Autodesk Fusion 360 part; units mm, degrees
(part 2 of 2)
  spline S18 degree 5 poles (-6.5449, 6.7429) (-6.5503, 6.7485) (-6.5613, 6.7594) (-6.5783, 6.7752) (-6.602, 6.7952) (-6.633, 6.8186) (-6.6649, 6.8409) (-6.6975, 6.8626) (-6.7305, 6.8839) (-6.7637, 6.905) (-6.7971, 6.9257) (-6.8309, 6.9462) (-6.8651, 6.9661) (-6.8998, 6.9854) (-6.9349, 7.0042) (-6.9705, 7.0225) (-7.0064, 7.0403) (-7.0427, 7.0577) (-7.0792, 7.0748) (-7.116, 7.0916) (-7.153, 7.108) (-7.1903, 7.1241) (-7.2279, 7.1398) (-7.2657, 7.1551) (-7.3038, 7.1701) (-7.3422, 7.1847) (-7.3809, 7.1989) (-7.4197, 7.2128) (-7.4588, 7.2264) (-7.4982, 7.2396) (-7.5377, 7.2526) (-7.5775, 7.2652) (-7.6174, 7.2774) (-7.6576, 7.2894) (-7.698, 7.301) (-7.7386, 7.3123) (-7.7793, 7.3233) (-7.8203, 7.334) (-7.8615, 7.3444) (-7.9028, 7.3544) (-7.9443, 7.3642) (-7.986, 7.3737) (-8.0279, 7.3828) (-8.07, 7.3916) (-8.1122, 7.4002) (-8.1545, 7.4084) (-8.1971, 7.4164) (-8.2398, 7.424) (-8.2826, 7.4313) (-8.3256, 7.4384) (-8.3688, 7.4451) (-8.4121, 7.4516) (-8.4555, 7.4577) (-8.4991, 7.4636) (-8.5429, 7.4692) (-8.5867, 7.4745) (-8.6307, 7.4795) (-8.6749, 7.4842) (-8.7191, 7.4886) (-8.7635, 7.4927) (-8.808, 7.4965) (-8.8527, 7.5001) (-8.8974, 7.5034) (-8.9423, 7.5063) (-8.9873, 7.509) (-9.0324, 7.5114) (-9.0777, 7.5136) (-9.123, 7.5154) (-9.1684, 7.5169) (-9.214, 7.5182) (-9.2596, 7.5192) (-9.2962, 7.5198) (-9.3237, 7.52) (-9.3421, 7.5202) (-9.3513, 7.5202) knots 0 0 0 0 0 0 0.01428571 0.02857143 0.04285714 0.05714286 0.07142857 0.08571429 0.1 0.11428571 0.12857143 0.14285714 0.15714286 0.17142857 0.18571429 0.2 0.21428571 0.22857143 0.24285714 0.25714286 0.27142857 0.28571429 0.3 0.31428571 0.32857143 0.34285714 0.35714286 0.37142857 0.38571429 0.4 0.41428571 0.42857143 0.44285714 0.45714286 0.47142857 0.48571429 0.5 0.51428571 0.52857143 0.54285714 0.55714286 0.57142857 0.58571429 0.6 0.61428571 0.62857143 0.64285714 0.65714286 0.67142857 0.68571429 0.7 0.71428571 0.72857143 0.74285714 0.75714286 0.77142857 0.78571429 0.8 0.81428571 0.82857143 0.84285714 0.85714286 0.87142857 0.88571429 0.9 0.91428571 0.92857143 0.94285714 0.95714286 0.97142857 0.98571429 1 1 1 1 1 1
  arc A38 (-9.3513, 7.5202) -> (-10.0419, 6.5697) centre (0, 0) ccw
  spline S19 degree 5 poles (-10.0419, 6.5697) (-10.039, 6.561) (-10.0332, 6.5436) (-10.0244, 6.5175) (-10.0126, 6.4829) (-9.9975, 6.4398) (-9.9822, 6.3968) (-9.9667, 6.3541) (-9.951, 6.3115) (-9.935, 6.2692) (-9.9187, 6.227) (-9.9023, 6.1851) (-9.8856, 6.1433) (-9.8686, 6.1017) (-9.8515, 6.0604) (-9.8341, 6.0192) (-9.8164, 5.9783) (-9.7986, 5.9376) (-9.7804, 5.897) (-9.7621, 5.8567) (-9.7435, 5.8166) (-9.7247, 5.7768) (-9.7056, 5.7371) (-9.6864, 5.6977) (-9.6668, 5.6585) (-9.6471, 5.6196) (-9.6271, 5.5808) (-9.6069, 5.5424) (-9.5864, 5.5041) (-9.5657, 5.4661) (-9.5448, 5.4283) (-9.5236, 5.3908) (-9.5022, 5.3536) (-9.4806, 5.3166) (-9.4587, 5.2799) (-9.4366, 5.2434) (-9.4142, 5.2072) (-9.3917, 5.1712) (-9.3688, 5.1356) (-9.3458, 5.1002) (-9.3225, 5.0651) (-9.299, 5.0303) (-9.2752, 4.9957) (-9.2511, 4.9615) (-9.2269, 4.9276) (-9.2024, 4.894) (-9.1776, 4.8607) (-9.1526, 4.8277) (-9.1274, 4.795) (-9.1019, 4.7627) (-9.0762, 4.7307) (-9.0502, 4.699) (-9.0239, 4.6678) (-8.9973, 4.6369) (-8.9705, 4.6064) (-8.9435, 4.5763) (-8.9162, 4.5465) (-8.8886, 4.517) (-8.8608, 4.4879) (-8.8328, 4.4593) (-8.8044, 4.4311) (-8.7757, 4.4035) (-8.7466, 4.3765) (-8.7171, 4.3501) (-8.6872, 4.3243) (-8.6571, 4.2989) (-8.6268, 4.2738) (-8.5964, 4.2491) (-8.5657, 4.2248) (-8.5346, 4.2013) (-8.5027, 4.179) (-8.4764, 4.1627) (-8.4561, 4.1514) (-8.4423, 4.1443) (-8.4354, 4.1409) knots -1 -1 -1 -1 -1 -1 -0.98571429 -0.97142857 -0.95714286 -0.94285714 -0.92857143 -0.91428571 -0.9 -0.88571429 -0.87142857 -0.85714286 -0.84285714 -0.82857143 -0.81428571 -0.8 -0.78571429 -0.77142857 -0.75714286 -0.74285714 -0.72857143 -0.71428571 -0.7 -0.68571429 -0.67142857 -0.65714286 -0.64285714 -0.62857143 -0.61428571 -0.6 -0.58571429 -0.57142857 -0.55714286 -0.54285714 -0.52857143 -0.51428571 -0.5 -0.48571429 -0.47142857 -0.45714286 -0.44285714 -0.42857143 -0.41428571 -0.4 -0.38571429 -0.37142857 -0.35714286 -0.34285714 -0.32857143 -0.31428571 -0.3 -0.28571429 -0.27142857 -0.25714286 -0.24285714 -0.22857143 -0.21428571 -0.2 -0.18571429 -0.17142857 -0.15714286 -0.14285714 -0.12857143 -0.11428571 -0.1 -0.08571429 -0.07142857 -0.05714286 -0.04285714 -0.02857143 -0.01428571 0 0 0 0 0 0
  line L19 (-8.4354, 4.1409) -> (-7.6212, 3.7403)
  arc A39 (-7.1196, 2.5104) -> (-7.6212, 3.7403) centre (-8.0626, 2.843) ccw
  circle A40 centre (0, 0) radius 17.5
  dimension "d9" = 35
  constraint concentric A0 A40
  measures "d9" diameter of A40
extrude "Extrude3" add sketch "Sketch1 (2)" along normal blind 7 contours A0 A1 L0 S0 A2 S1 L1 A3 A4 A5 L2 S2 A6 S3 L3 A7 A8 A9 L4 S4 A10 S5 L5 A11 A12 A13 L6 S6 A14 S7 L7 A15 A16 A17 L8 S8 A18 S9 L9 A19 A20 A21 L10 S10 A22 S11 L11 A23 A24 A25 L12 S12 A26 S13 L13 A27 A28 A29 L14 S14 A30 S15 L15 A31 A32 A33 L16 S16 A34 S17 L17 A35 A36 A37 L18 S18 A38 S19 L19 A39 | A40 bodies 1 in component "Spur Gear (10 teeth)"
sketch "Sketch2 (2)" plane through (0, 0, 38) normal (0, 0, 1) x (-1, 0, 0)
  line L0 (-3.5, -6.0622) -> (3.5, -6.0622)
  line L1 (3.5, -6.0622) -> (7, 0)
  line L2 (7, 0) -> (3.5, 6.0622)
  line L3 (3.5, 6.0622) -> (-3.5, 6.0622)
  line L4 (-3.5, 6.0622) -> (-7, 0)
  line L5 (-7, 0) -> (-3.5, -6.0622)
  circle A0 centre (0, 0) radius 5.75
extrude "Extrude4" cut sketch "Sketch2 (2)" against normal blind 31 contours L0 L1 L2 L3 L4 L5 | A0 bodies 1 in component "Spur Gear (10 teeth)"
extrude "Extrude5" cut 1 faces at (-2.3777, 0.694, 0) along direction (0, 0, 1) blind 7 on bodies 1 bodies 1 in component "Spur Gear (10 teeth)"
extrude "Extrude6" add 1 faces at (8.7557, 4.5517, 14) along direction (0, 0, 1) blind 2 on bodies 1 bodies 1 in component "Spur Gear (10 teeth)"
sketch "Sketch3 (2)" plane through (0, 0, 7) normal (0, 0, -1) x (1, 0, 0)
  line L0 (-3.5, 6.0622) -> (3.5, 6.0622)
  line L1 (3.5, 6.0622) -> (7, 0)
  line L2 (7, 0) -> (3.5, -6.0622)
  line L3 (3.5, -6.0622) -> (-3.5, -6.0622)
  line L4 (-3.5, -6.0622) -> (-7, 0)
  line L5 (-7, 0) -> (-3.5, 6.0622)
  circle A0 centre (0, 0) radius 17.5
  arc A1 (-44.2503, 36.7173) -> (-43.1721, 30.6989) centre (-41.1721, 34.163) ccw
  line L6 (-26.1836, 58.9803) -> (-29.7874, 57.2447)
  line L7 (-37.9866, 52.1658) -> (-38.2509, 52.5535)
  line L8 (7.3412, 1.535) -> (14.1913, -2.4199)
  arc A2 (44.2503, 36.7173) -> (-44.2503, 36.7173) centre (0, 0) ccw
  arc A3 (-2.3412, -7.1252) -> (2.3412, -7.1252) centre (0, 0) ccw
  line L9 (17.1006, -62.224) -> (20.9229, -61.0449)
  line L10 (37.9866, 52.1658) -> (34.6817, 54.419)
  arc A4 (57.265, -30.7526) -> (59.7475, -25.5977) centre (0, 0) ccw
  line L11 (-7.6356, -64.0777) -> (-7.7055, -64.5417)
  line L12 (-34.6817, -54.419) -> (-34.946, -54.8067)
  arc A5 (2, -64.9692) -> (7.7055, -64.5417) centre (0, 0) ccw
  arc A6 (-48.1721, 22.0387) -> (-53.9232, 19.9633) centre (-50.1721, 18.5746) ccw
  line L13 (56.8586, 30.5179) -> (54.8586, 33.9821)
  arc A7 (55.265, 34.2167) -> (52.042, 38.944) centre (0, 0) ccw
  arc A8 (9.1913, -11.0801) -> (14.6554, -9.616) centre (11.1913, -7.616) ccw
  line L14 (-38.2509, -52.5535) -> (-37.9866, -52.1658)
  arc A9 (64.6381, 6.8496) -> (63.7854, 12.5072) centre (0, 0) ccw
  line L15 (29.7874, -57.2447) -> (29.991, -57.6675)
  line L16 (42.405, -48.6422) -> (45.3372, -45.9215)
  line L17 (-45.6564, -46.2655) -> (-45.3372, -45.9215)
  line L18 (52.042, 38.944) -> (51.6751, 38.6514)
  line L19 (-29.7874, -57.2447) -> (-26.1836, -58.9803)
  line L20 (64.1702, 6.8145) -> (64.6381, 6.8496)
  line L21 (-26.1836, -58.9803) -> (-26.3872, -59.403)
  arc A10 (5, -52.7376) -> (9.6729, -56.6806) centre (9, -52.7376) ccw
  line L22 (51.6751, -38.6514) -> (52.042, -38.944)
  line L23 (-54.8586, -33.9821) -> (-55.265, -34.2167)
  line L24 (15.6554, -7.884) -> (14.6554, -9.616)
  arc A11 (21.0612, -61.4933) -> (26.3872, -59.403) centre (0, 0) ccw
  line L25 (-54.8586, 33.9821) -> (-56.8586, 30.5179)
  line L26 (-11.6608, -63.9455) -> (-11.5909, -63.4815)
  arc A12 (-42.7242, -48.9862) -> (-38.2509, -52.5535) centre (0, 0) ccw
  line L27 (-42.405, -48.6422) -> (-42.7242, -48.9862)
  arc A13 (-49.548, -42.0713) -> (-45.6564, -46.2655) centre (0, 0) ccw
  line L28 (49.1812, 41.7788) -> (49.548, 42.0713)
  line L29 (-37.9866, -52.1658) -> (-34.6817, -54.419)
  arc A14 (-23.6426, 19.4236) -> (-18.8944, 19.9813) centre (-21.6426, 22.8877) ccw
  line L30 (2, -64.5) -> (2, -64.9692)
  arc A15 (-9.6729, -56.6806) -> (-5, -52.7376) centre (-9, -52.7376) ccw
  line L31 (26.1836, -58.9803) -> (29.7874, -57.2447)
  arc A16 (-17.2389, -62.6723) -> (-11.6608, -63.9455) centre (0, 0) ccw
  arc A17 (-34.946, -54.8067) -> (-29.991, -57.6675) centre (0, 0) ccw
  line L32 (-49.1812, -41.7788) -> (-49.548, -42.0713)
  arc A18 (52.042, -38.944) -> (55.265, -34.2167) centre (0, 0) ccw
  arc A19 (43.1721, 30.6989) -> (44.2503, 36.7173) centre (41.1721, 34.163) ccw
  arc A20 (61.2088, -21.8742) -> (62.8953, -16.4069) centre (0, 0) ccw
  arc A21 (62.8953, 16.4069) -> (61.2088, 21.8742) centre (0, 0) ccw
  line L33 (59.3107, -25.4262) -> (60.772, -21.7027)
  line L34 (5, -52.7376) -> (5, -30.1869)
  line L35 (61.2088, 21.8742) -> (60.772, 21.7027)
  line L36 (17.2389, -62.6723) -> (17.1006, -62.224)
  line L37 (7.7055, -64.5417) -> (7.6356, -64.0777)
  line L38 (64.6381, -6.8496) -> (64.1702, -6.8145)
  line L39 (42.405, 48.6422) -> (42.7242, 48.9862)
  line L40 (45.3372, -45.9215) -> (45.6564, -46.2655)
  arc A22 (-7.7055, -64.5417) -> (-2, -64.9692) centre (0, 0) ccw
  line L41 (64.1702, -6.8145) -> (64.4691, -2.8257)
  line L42 (62.8953, -16.4069) -> (62.4378, -16.3025)
  arc A23 (7.8571, -26.3537) -> (5, -30.1869) centre (9, -30.1869) ccw
  line L43 (62.4378, -16.3025) -> (63.3279, -12.4027)
  line L44 (-63.7854, -12.5072) -> (-63.3279, -12.4027)
  arc A24 (5, 13.5) -> (1, 17.5) centre (1, 13.5) ccw
  line L45 (26.1836, 58.9803) -> (26.3872, 59.403)
  line L46 (20.9229, -61.0449) -> (21.0612, -61.4933)
  arc A25 (26.3872, 59.403) -> (21.0612, 61.4933) centre (0, 0) ccw
  line L47 (-34.6817, 54.419) -> (-37.9866, 52.1658)
  arc A26 (-57.265, 30.7526) -> (-59.7475, 25.5977) centre (0, 0) ccw
  arc A27 (-62.8953, -16.4069) -> (-61.2088, -21.8742) centre (0, 0) ccw
  line L48 (-64.937, -2.8607) -> (-64.4691, -2.8257)
  arc A28 (-64.6381, -6.8496) -> (-63.7854, -12.5072) centre (0, 0) ccw
  line L49 (-23.6426, 19.4236) -> (-43.1721, 30.6989)
  line L50 (64.4691, 2.8257) -> (64.1702, 6.8145)
  arc A29 (-63.7854, 12.5072) -> (-64.6381, 6.8496) centre (0, 0) ccw
  arc A30 (-61.2088, 21.8742) -> (-62.8953, 16.4069) centre (0, 0) ccw
  arc A31 (29.991, -57.6675) -> (34.946, -54.8067) centre (0, 0) ccw
  arc A32 (15.6554, -7.884) -> (14.1913, -2.4199) centre (12.1913, -5.884) ccw
  line L51 (2, 64.9692) -> (2, 64.5)
  arc A33 (28.6426, 10.7633) -> (26.7515, 6.3723) centre (30.6426, 7.2992) ccw
  line L52 (5, 13.5) -> (5, 5.5902)
  line L53 (-63.3279, -12.4027) -> (-62.4378, -16.3025)
  line L54 (62.4378, 16.3025) -> (62.8953, 16.4069)
  line L55 (42.7242, -48.9862) -> (42.405, -48.6422)
  line L56 (-26.3872, 59.403) -> (-26.1836, 58.9803)
  arc A34 (7.7055, 64.5417) -> (2, 64.9692) centre (0, 0) ccw
  arc A35 (34.946, 54.8067) -> (29.991, 57.6675) centre (0, 0) ccw
  line L57 (21.0612, 61.4933) -> (20.9229, 61.0449)
  line L58 (7.6356, -64.0777) -> (11.5909, -63.4815)
  line L59 (55.265, -34.2167) -> (54.8586, -33.9821)
  line L60 (-62.4378, 16.3025) -> (-63.3279, 12.4027)
  line L61 (-20.9229, -61.0449) -> (-17.1006, -62.224)
  line L62 (-62.8953, 16.4069) -> (-62.4378, 16.3025)
  arc A36 (-38.2509, 52.5535) -> (-42.7242, 48.9862) centre (0, 0) ccw
  line L63 (-52.042, -38.944) -> (-51.6751, -38.6514)
  line L64 (-63.3279, 12.4027) -> (-63.7854, 12.5072)
  line L65 (-55.265, 34.2167) -> (-54.8586, 33.9821)
  line L66 (-56.8586, 30.5179) -> (-57.265, 30.7526)
  line L67 (49.1812, -41.7788) -> (51.6751, -38.6514)
  line L68 (-61.2088, -21.8742) -> (-60.772, -21.7027)
  line L69 (-64.4691, -2.8257) -> (-64.1702, -6.8145)
  line L70 (-17.1006, -62.224) -> (-17.2389, -62.6723)
  arc A37 (-5, -30.1869) -> (-7.8571, -26.3537) centre (-9, -30.1869) ccw
  line L71 (-2.3412, -7.1252) -> (-9.1913, -11.0801)
  line L72 (-29.991, -57.6675) -> (-29.7874, -57.2447)
  line L73 (43.1721, 30.6989) -> (23.6426, 19.4236)
  line L74 (-49.548, 42.0713) -> (-49.1812, 41.7788)
  arc A38 (-26.3872, -59.403) -> (-21.0612, -61.4933) centre (0, 0) ccw
  line L75 (11.5909, -63.4815) -> (11.6608, -63.9455)
  line L76 (11.6608, 63.9455) -> (11.5909, 63.4815)
  line L77 (-48.1721, 22.0387) -> (-28.6426, 10.7633)
  line L78 (56.8586, -30.5179) -> (57.265, -30.7526)
  line L79 (-62.4378, -16.3025) -> (-62.8953, -16.4069)
  line L80 (-64.1702, -6.8145) -> (-64.6381, -6.8496)
  line L81 (7.6356, 64.0777) -> (7.7055, 64.5417)
  line L82 (9.1913, -11.0801) -> (2.3412, -7.1252)
  line L83 (-51.6751, -38.6514) -> (-49.1812, -41.7788)
  arc A39 (-53.9232, 19.9633) -> (-9.6729, -56.6806) centre (0, 0) ccw
  line L84 (-14.1913, -2.4199) -> (-7.3412, 1.535)
  arc A40 (-64.937, 2.8607) -> (-64.937, -2.8607) centre (0, 0) ccw
  line L85 (-2, 64.5) -> (-2, 64.9692)
  line L86 (20.9229, 61.0449) -> (17.1006, 62.224)
  line L87 (-60.772, -21.7027) -> (-59.3107, -25.4262)
  arc A41 (-2, 64.9692) -> (-7.7055, 64.5417) centre (0, 0) ccw
  arc A42 (17.2389, 62.6723) -> (11.6608, 63.9455) centre (0, 0) ccw
  arc A43 (-55.265, -34.2167) -> (-52.042, -38.944) centre (0, 0) ccw
  line L88 (-59.7475, 25.5977) -> (-59.3107, 25.4262)
  arc A44 (-29.991, 57.6675) -> (-34.946, 54.8067) centre (0, 0) ccw
  arc A45 (64.937, -2.8607) -> (64.937, 2.8607) centre (0, 0) ccw
  line L89 (64.4691, -2.8257) -> (64.937, -2.8607)
  line L90 (-45.3372, -45.9215) -> (-42.405, -48.6422)
  line L91 (57.265, 30.7526) -> (56.8586, 30.5179)
  line L92 (63.3279, 12.4027) -> (62.4378, 16.3025)
  line L93 (34.6817, 54.419) -> (34.946, 54.8067)
  line L94 (60.772, -21.7027) -> (61.2088, -21.8742)
  line L95 (45.6564, 46.2655) -> (45.3372, 45.9215)
  line L96 (54.8586, -33.9821) -> (56.8586, -30.5179)
  line L97 (26.3872, -59.403) -> (26.1836, -58.9803)
  line L98 (45.3372, 45.9215) -> (42.405, 48.6422)
  arc A46 (49.548, 42.0713) -> (45.6564, 46.2655) centre (0, 0) ccw
  line L99 (64.937, 2.8607) -> (64.4691, 2.8257)
  arc A47 (11.6608, -63.9455) -> (17.2389, -62.6723) centre (0, 0) ccw
  arc A48 (38.2509, -52.5535) -> (42.7242, -48.9862) centre (0, 0) ccw
  arc A49 (45.6564, -46.2655) -> (49.548, -42.0713) centre (0, 0) ccw
  line L100 (34.6817, -54.419) -> (37.9866, -52.1658)
  line L101 (38.2509, 52.5535) -> (37.9866, 52.1658)
  line L102 (37.9866, -52.1658) -> (38.2509, -52.5535)
  arc A50 (53.9232, 19.9633) -> (48.1721, 22.0387) centre (50.1721, 18.5746) ccw
  arc A51 (63.7854, -12.5072) -> (64.6381, -6.8496) centre (0, 0) ccw
  arc A52 (42.7242, 48.9862) -> (38.2509, 52.5535) centre (0, 0) ccw
  line L103 (63.7854, 12.5072) -> (63.3279, 12.4027)
  arc A53 (59.7475, 25.5977) -> (57.265, 30.7526) centre (0, 0) ccw
  line L104 (59.7475, -25.5977) -> (59.3107, -25.4262)
  line L105 (60.772, 21.7027) -> (59.3107, 25.4262)
  line L106 (49.548, -42.0713) -> (49.1812, -41.7788)
  line L107 (63.3279, -12.4027) -> (63.7854, -12.5072)
  line L108 (34.946, -54.8067) -> (34.6817, -54.419)
  line L109 (51.6751, 38.6514) -> (49.1812, 41.7788)
  line L110 (59.3107, 25.4262) -> (59.7475, 25.5977)
  line L111 (54.8586, 33.9821) -> (55.265, 34.2167)
  arc A54 (-45.6564, 46.2655) -> (-49.548, 42.0713) centre (0, 0) ccw
  arc A55 (-21.0612, 61.4933) -> (-26.3872, 59.403) centre (0, 0) ccw
  arc A56 (-52.042, 38.944) -> (-55.265, 34.2167) centre (0, 0) ccw
  arc A57 (18.8944, 19.9813) -> (23.6426, 19.4236) centre (21.6426, 22.8877) ccw
  line L112 (-34.946, 54.8067) -> (-34.6817, 54.419)
  line L113 (-42.405, 48.6422) -> (-45.3372, 45.9215)
  line L114 (11.5909, 63.4815) -> (7.6356, 64.0777)
  arc A58 (18.8944, 19.9813) -> (-18.8944, 19.9813) centre (0, 0) ccw
  line L115 (-51.6751, 38.6514) -> (-52.042, 38.944)
  line L116 (-29.7874, 57.2447) -> (-29.991, 57.6675)
  arc A59 (9.6729, -56.6806) -> (53.9232, 19.9633) centre (0, 0) ccw
  line L117 (2, 64.5) -> (-2, 64.5)
  line L118 (-2, -64.5) -> (2, -64.5)
  line L119 (-1, 17.5) -> (1, 17.5)
  arc A60 (-26.7515, 6.3723) -> (-7.8571, -26.3537) centre (0, 0) ccw
  line L120 (-49.1812, 41.7788) -> (-51.6751, 38.6514)
  arc A61 (7.8571, -26.3537) -> (26.7515, 6.3723) centre (0, 0) ccw
  line L121 (-64.6381, 6.8496) -> (-64.1702, 6.8145)
  arc A62 (-5, 5.5902) -> (-7.3412, 1.535) centre (0, 0) ccw
  line L122 (-5, -30.1869) -> (-5, -52.7376)
  line L123 (17.1006, 62.224) -> (17.2389, 62.6723)
  line L124 (-7.7055, 64.5417) -> (-7.6356, 64.0777)
  line L125 (-20.9229, 61.0449) -> (-21.0612, 61.4933)
  arc A63 (-14.6554, -9.616) -> (-9.1913, -11.0801) centre (-11.1913, -7.616) ccw
  line L126 (29.991, 57.6675) -> (29.7874, 57.2447)
  line L127 (-14.6554, -9.616) -> (-15.6554, -7.884)
  line L128 (-42.7242, 48.9862) -> (-42.405, 48.6422)
  arc A64 (-14.1913, -2.4199) -> (-15.6554, -7.884) centre (-12.1913, -5.884) ccw
  line L129 (-59.3107, -25.4262) -> (-59.7475, -25.5977)
  line L130 (-17.1006, 62.224) -> (-20.9229, 61.0449)
  line L131 (-64.1702, 6.8145) -> (-64.4691, 2.8257)
  line L132 (-5, 5.5902) -> (-5, 13.5)
  line L133 (29.7874, 57.2447) -> (26.1836, 58.9803)
  line L134 (-11.5909, -63.4815) -> (-7.6356, -64.0777)
  arc A65 (-59.7475, -25.5977) -> (-57.265, -30.7526) centre (0, 0) ccw
  arc A66 (7.3412, 1.535) -> (5, 5.5902) centre (0, 0) ccw
  line L135 (-11.5909, 63.4815) -> (-11.6608, 63.9455)
  line L136 (-57.265, -30.7526) -> (-56.8586, -30.5179)
  line L137 (-45.3372, 45.9215) -> (-45.6564, 46.2655)
  line L138 (-59.3107, 25.4262) -> (-60.772, 21.7027)
  line L139 (-21.0612, -61.4933) -> (-20.9229, -61.0449)
  line L140 (-60.772, 21.7027) -> (-61.2088, 21.8742)
  line L141 (-2, -64.9692) -> (-2, -64.5)
  line L142 (28.6426, 10.7633) -> (48.1721, 22.0387)
  arc A67 (-1, 17.5) -> (-5, 13.5) centre (-1, 13.5) ccw
  line L143 (-56.8586, -30.5179) -> (-54.8586, -33.9821)
  line L144 (-17.2389, 62.6723) -> (-17.1006, 62.224)
  arc A68 (-26.7515, 6.3723) -> (-28.6426, 10.7633) centre (-30.6426, 7.2992) ccw
  arc A69 (-11.6608, 63.9455) -> (-17.2389, 62.6723) centre (0, 0) ccw
  line L145 (-7.6356, 64.0777) -> (-11.5909, 63.4815)
  line L146 (-64.4691, 2.8257) -> (-64.937, 2.8607)
extrude "Extrude1'" add sketch "Sketch3 (2)" along normal blind 6 separate body contours L0 L1 L2 L3 L4 L5 | A0 L8 A24 A32 L52 A66 | A0 L8 A3 A8 A24 A32 L52 L71 L82 L84 A62 A63 A64 L132 A66 A67 | A0 L84 A62 A64 L132 A67 | A0 A3 A8 L71 L82 A63 | L6 L7 L9 L10 A4 L11 L12 A5 L13 A7 L14 A9 L15 L16 L17 L18 L19 L20 L21 L22 L23 A11 L25 L26 A12 L27 A13 L28 L29 L30 L31 A16 A17 L32 A18 A20 A21 L33 L35 L36 L37 L38 L39 L40 A22 L41 L42 L43 L44 L45 L46 A25 L47 A26 A27 L48 A28 L50 A29 A30 A31 L51 L53 L54 L55 L56 A34 A35 L57 L58 L59 L60 L61 L62 A36 L63 L64 L65 L66 L67 L68 L69 L70 L72 L74 A38 L75 L76 L78 L79 L80 L81 L83 A40 L85 L86 L87 A41 A42 A43 L88 A44 A45 L89 L90 L91 L92 L93 L94 L95 L96 L97 L98 A46 L99 A47 A48 A49 L100 L101 L102 A51 A52 L103 A53 L104 L105 L106 L107 L108 L109 L110 L111 A54 A55 A56 L112 L113 L114 L115 L116 L117 L118 L120 L121 L123 L124 L125 L126 L128 L129 L130 L131 L133 L134 A65 L135 L136 L137 L138 L139 L140 L141 L143 L144 A69 L145 L146 makes body 2
chamfer "Chamfer1" distance 2 angle 45 1 edges at (16.3157, 6.3283, 16) on bodies 1 in component "Spur Gear (10 teeth)"
component "Spur Gear (10 teeth)" placed x (1, 0, 0) y (0, 1, 0) z (0, 0, 1) at (0, 0, 0)
